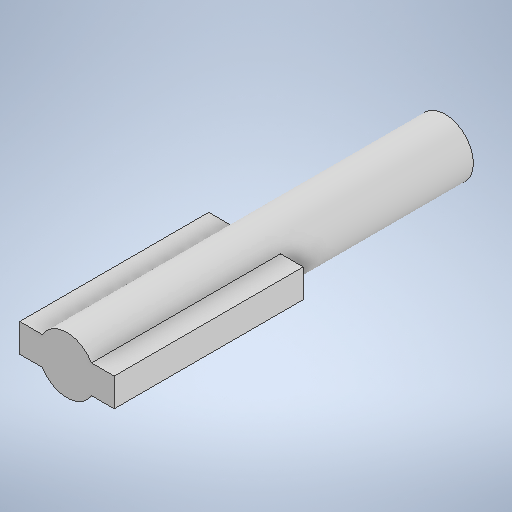
# Autodesk Inventor part: Pin
Saved by Autodesk Inventor 2025.4 (Build 294407000, 407)
## iProperties
Created: 2026-03-08
Part Number: Pin
Material: Generic
Document SubType Name: Modeling
Designer: Amir
Density: 1 g/cm^3
Appearance: Default
Author: Amir
Autodesk Inventor part; units mm, degrees
ref_plane "YZ Plane" through (0, 0, 0) normal (1, 0, 0) x (0, 1, 0)
ref_plane "XZ Plane" through (0, 0, 0) normal (0, 1, 0) x (-1, 0, 0)
ref_plane "XY Plane" through (0, 0, 0) normal (0, 0, 1) x (1, 0, 0)
sketch "Sketch1" plane through (0, 0, 0) normal (0, 0, 1) x (1, 0, 0)
  line L0 (2.5, -0.75) -> (2.5, 0.75)
  line L1 (-2.5, 0.75) -> (-2.5, -0.75)
  line L2 (2.5, 0.75) -> (1.299, 0.75)
  line L3 (-1.299, 0.75) -> (-2.5, 0.75)
  line L4 (-2.5, -0.75) -> (-1.299, -0.75)
  line L5 (1.299, -0.75) -> (2.5, -0.75)
  circle A0 centre (0, 0) radius 1.5
  dimension "d5" = 3
  dimension "d0" = 5
  dimension "d1" = 1.5
  dimension "d4" = 1.5
  dimension "d6" = 0.75
  dimension "d7" = 0.75
  dimension "d8" = 2.5
  constraints: 12 end point, 5 parallel, 2 horizontal, 2 perpendicular, 1 coincident, 3 other
  measures "d0" distance of L1.start L0.end
  measures "d1" distance of L5.end L0.end
  measures "d4" distance between parallel lines of L3 L4
  measures "d6" distance from line of point (0, 0) L2
  measures "d7" distance from line of point (0, 0) L4
  measures "d8" distance from line of L1 point (0, 0)
extrude "Extrusion1" add sketch "Sketch1" against normal blind 10 contours A0
extrude "Extrusion2" add sketch "Sketch1" along normal blind 10
body "Solid1"
